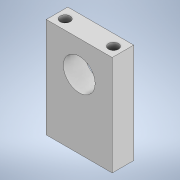
# Autodesk Inventor part: Wrist Support
Saved by Autodesk Inventor 2022 (Build 260153000, 153)
## iProperties
Created: 2022-03-11
Part Number: Wrist Support
Material: Generic
Document SubType Name: Modeling
Designer: legob
Density: 1 g/cm^3
Appearance: Default
Author: legob
Autodesk Inventor part; units mm, degrees
ref_plane "YZ Plane" through (0, 0, 0) normal (1, 0, 0) x (0, 1, 0)
ref_plane "XZ Plane" through (0, 0, 0) normal (0, 1, 0) x (-1, 0, 0)
ref_plane "XY Plane" through (0, 0, 0) normal (0, 0, 1) x (1, 0, 0)
sketch "Sketch1" plane through (0, 0, 0) normal (0, 0, 1) x (1, 0, 0)
  circle A0 centre (22.919, 29.5195) radius 18.75
  line L0 (-15.9938, 66.3532) -> (61.8383, 66.3532)
  line L1 (61.8383, 66.3532) -> (61.8383, -51.7605)
  line L2 (61.8383, -51.7605) -> (-15.9938, -51.7605)
  line L3 (-15.9938, -51.7605) -> (-15.9938, 66.3532)
  point P0 (0, 0)
  dimension "d0" = 37.5
  dimension "d1" = 77.8321
  dimension "d2" = 118.1137
  dimension "d3" = 38.9128
  dimension "d4" = 81.28
  constraints: 8 end point, 2 parallel, 1 centre point, 1 horizontal, 1 perpendicular
  measures "d0" diameter of A0
  measures "d1" distance of L0.start L0.end
  measures "d2" distance of L2.end L0.start
  measures "d3" distance from line of L3 A0.centre
  measures "d4" distance from line of L2 A0.centre
extrude "Extrusion1" add sketch "Sketch1" along normal blind 25.4
sketch "Sketch2" plane through (-15.9938, 66.3532, 0) normal (0, 1, 0) x (1, 0, 0)
  point P0 (15.9938, 0)
  point P1 (10.6081, -13.72)
hole "Hole1" at (-5.3858, 66.3532, 13.72) direction (0, -1, 0) diameter 8.4328 end through all counterbore diameter 11.9062 counterbore depth 7.9502 clearance for "Socket Head Cap Screw" size "5/16" standard "Ansi Unified Screw Threads"
sketch "Sketch3" plane through (-15.9938, 66.3532, 0) normal (0, 1, 0) x (1, 0, 0)
  point P0 (15.9938, 0)
  point P1 (67.1861, -13.2652)
hole "Hole2" at (51.1923, 66.3532, 13.2652) direction (0, -1, 0) diameter 8.4328 end through all counterbore diameter 11.9062 counterbore depth 7.9502 clearance for "Socket Head Cap Screw" size "5/16" standard "Ansi Unified Screw Threads"
body "Solid1"
